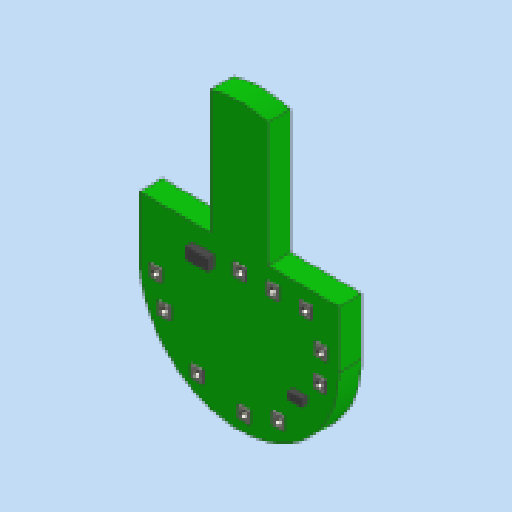
# Autodesk Inventor part: Sensor_PCB
Saved by Autodesk Inventor 2024 (Build 280153000, 153)
## iProperties
Created: 2025-02-15
Part Number: Sensor_PCB
Material: Generic
Document SubType Name: Modeling
Designer: XxPan
Density: 1 g/cm^3
Appearance: Default
Author: XxPan
Autodesk Inventor part; units mm, degrees
ref_plane "YZ Plane" through (0, 0, 0) normal (1, 0, 0) x (0, 1, 0)
ref_plane "XZ Plane" through (0, 0, 0) normal (0, 1, 0) x (-1, 0, 0)
ref_plane "XY Plane" through (0, 0, 0) normal (0, 0, 1) x (1, 0, 0)
sketch "Sketch1" plane through (0, 0, 0) normal (0, 0, 1) x (-1, 0, 0)
  line L0 (0, 0) -> (0, 6) construction
  line L1 (7, 0) -> (7, 6)
  line L2 (-7, 6) -> (-7, 0)
  arc A0 (-7, 0) -> (7, 0) centre (0, 0) ccw
  arc A1 (7, 6) -> (-7, 6) centre (0, 6) ccw
  point P0 (0, 3)
  dimension "d4" = 6
  dimension "d5" = 14
  constraints: 8 end point, 4 point on circle, 4 tangent, 2 centre point, 1 midpoint, 1 parallel, 1 vertical
  measures "d4" distance of L0.start L0.end
  measures "d5" diameter of A1
extrude "Extrusion1" add sketch "Sketch1" along normal blind 1.6
sketch "Sketch2" plane through (0, 0, 0) normal (0, 0, -1) x (-1, 0, 0)
  line L0 (-7, -6) -> (-7, 0) projected
  line L1 (-7, -2) -> (-2, -2)
  line L2 (-2, -2) -> (-2, 6.7082)
  arc A0 (7, 0) -> (-7, 0) centre (0, 0) ccw projected
  line L3 (7, -2) -> (2, -2)
  line L4 (2, -2) -> (2, 6.7082)
  line L5 (7, 0) -> (7, -6) projected
  line L6 (0, -17) -> (0, 11) construction
  line L7 (-9.8, 0) -> (9.8, 0) construction
  dimension "d6" = 4
  dimension "d7" = 2
  constraints: 8 end point, 3 point on line, 2 perpendicular, 2 point on circle, 1 horizontal, 1 other
  measures "d6" distance between parallel lines of L4 L2
  measures "d7" distance between parallel lines of L7 L1
extrude "Extrusion2" cut sketch "Sketch2" against normal up to surface (1.6 mm away)
sketch "Sketch5" plane through (0, 0, 1.6) normal (0, 0, 1) x (1, 0, 0)
  line L0 (-0.325, -2.875) -> (0.525, -2.875)
  line L1 (0.525, -2.875) -> (0.525, -3.725)
  line L2 (0.525, -3.725) -> (-0.325, -3.725)
  line L3 (-0.325, -3.725) -> (-0.325, -2.875)
  line L4 (1.975, -2.875) -> (2.825, -2.875)
  line L5 (2.825, -2.875) -> (2.825, -3.725)
  line L6 (2.825, -3.725) -> (1.975, -3.725)
  line L7 (1.975, -3.725) -> (1.975, -2.875)
  line L8 (4.275, -2.875) -> (5.125, -2.875)
  line L9 (5.125, -2.875) -> (5.125, -3.725)
  line L10 (5.125, -3.725) -> (4.275, -3.725)
  line L11 (4.275, -3.725) -> (4.275, -2.875)
  line L12 (5.375, -4.875) -> (6.225, -4.875)
  line L13 (6.225, -4.875) -> (6.225, -5.725)
  line L14 (6.225, -5.725) -> (5.375, -5.725)
  line L15 (5.375, -5.725) -> (5.375, -4.875)
  line L16 (5.275, -6.875) -> (6.125, -6.875)
  line L17 (6.125, -6.875) -> (6.125, -7.725)
  line L18 (6.125, -7.725) -> (5.275, -7.725)
  line L19 (5.275, -7.725) -> (5.275, -6.875)
  line L20 (2.375, -10.575) -> (3.225, -10.575)
  line L21 (3.225, -10.575) -> (3.225, -11.425)
  line L22 (3.225, -11.425) -> (2.375, -11.425)
  line L23 (2.375, -11.425) -> (2.375, -10.575)
  line L24 (-0.025, -11.375) -> (0.825, -11.375)
  line L25 (0.825, -11.375) -> (0.825, -12.225)
  line L26 (0.825, -12.225) -> (-0.025, -12.225)
  line L27 (-0.025, -12.225) -> (-0.025, -11.375)
  line L28 (-3.325, -10.575) -> (-2.475, -10.575)
  line L29 (-2.475, -10.575) -> (-2.475, -11.425)
  line L30 (-2.475, -11.425) -> (-3.325, -11.425)
  line L31 (-3.325, -11.425) -> (-3.325, -10.575)
  line L32 (-5.625, -7.875) -> (-4.775, -7.875)
  line L33 (-4.775, -7.875) -> (-4.775, -8.725)
  line L34 (-4.775, -8.725) -> (-5.625, -8.725)
  line L35 (-5.625, -8.725) -> (-5.625, -7.875)
  line L36 (-6.225, -5.875) -> (-5.375, -5.875)
  line L37 (-5.375, -5.875) -> (-5.375, -6.725)
  line L38 (-5.375, -6.725) -> (-6.225, -6.725)
  line L39 (-6.225, -6.725) -> (-6.225, -5.875)
  line L40 (7, -6) -> (7, -2) projected
  line L41 (7, -2) -> (2, -2) projected
  point P0 (0, 0)
  point P1 (4.7, -2.875)
  point P2 (5.125, -3.3)
  dimension "d22" = 0.85
  dimension "d23" = 0.85
  dimension "d24" = 0.85
  dimension "d25" = 0.85
  dimension "d26" = 0.85
  dimension "d27" = 0.85
  dimension "d28" = 0.85
  dimension "d29" = 0.85
  dimension "d30" = 0.85
  dimension "d31" = 0.85
  dimension "d32" = 0.85
  dimension "d33" = 0.85
  dimension "d34" = 0.85
  dimension "d35" = 0.85
  dimension "d36" = 0.85
  dimension "d37" = 0.85
  dimension "d38" = 0.85
  dimension "d39" = 0.85
  dimension "d40" = 0.85
  dimension "d41" = 0.85
  dimension "d42" = 2.3
  dimension "d43" = 2.3
  dimension "d44" = 2
  dimension "d45" = 2
  dimension "d46" = 0.8
  dimension "d47" = 2.4
  dimension "d48" = 0.1
  dimension "d49" = 2.3
  dimension "d50" = 1.3
  dimension "d51" = 1.1
  dimension "d52" = 2.9
  dimension "d53" = 3.7
  dimension "d54" = 0.8
  dimension "d55" = 3.3
  dimension "d56" = 2.3
  dimension "d57" = 2.7
  dimension "d58" = 0.6
  dimension "d59" = 2
  constraints: 80 end point, 20 parallel, 10 horizontal, 10 perpendicular, 2 collinear, 2 midpoint
  measures "d22" distance of L1.end L2.end
  measures "d23" distance of L0.end L1.end
  measures "d24" distance of L5.end L6.end
  measures "d25" distance of L4.end L5.end
  measures "d26" distance of L9.end L10.end
  measures "d27" distance of L8.end L9.end
  measures "d28" distance of L13.end L14.end
  measures "d29" distance of L12.end L13.end
  measures "d30" distance of L17.end L18.end
  measures "d31" distance of L16.end L17.end
  measures "d32" distance of L21.end L22.end
  measures "d33" distance of L20.end L21.end
  measures "d34" distance of L25.end L26.end
  measures "d35" distance of L24.end L25.end
  measures "d36" distance of L29.end L30.end
  measures "d37" distance of L28.end L29.end
  measures "d38" distance of L33.end L34.end
  measures "d39" distance of L32.end L33.end
  measures "d40" distance of L37.end L38.end
  measures "d41" distance of L36.end L37.end
  measures "d42" distance between parallel lines of L5 L1
  measures "d43" distance between parallel lines of L9 L5
  measures "d44" distance between parallel lines of L14 L10
  measures "d45" distance between parallel lines of L18 L14
  measures "d46" distance between parallel lines of L20 L24
  measures "d47" distance between parallel lines of L21 L25
  measures "d48" distance between parallel lines of L17 L13
  measures "d49" distance from line of L40 point (4.7, -2.875)
  measures "d50" distance from line of L41 point (5.125, -3.3)
  measures "d51" distance between parallel lines of L13 L9
  measures "d52" distance between parallel lines of L17 L21
  measures "d53" distance between parallel lines of L16 L20
  measures "d54" distance between parallel lines of L26 L30
  measures "d55" distance between parallel lines of L27 L31
  measures "d56" distance between parallel lines of L35 L31
  measures "d57" distance between parallel lines of L28 L32
  measures "d58" distance between parallel lines of L35 L39
  measures "d59" distance between parallel lines of L32 L36
extrude "Extrusion5" add sketch "Sketch5" along normal blind 0.1 and the other way blind 1.7
sketch "Sketch6" plane through (0, 0, 1.7) normal (0, 0, 1) x (1, 0, 0)
  line L0 (0.525, -2.875) -> (-0.325, -2.875) projected
  line L1 (2.825, -2.875) -> (1.975, -2.875) projected
  line L2 (5.125, -2.875) -> (4.275, -2.875) projected
  line L3 (6.225, -4.875) -> (5.375, -4.875) projected
  line L4 (6.125, -6.875) -> (5.275, -6.875) projected
  line L5 (3.225, -10.575) -> (2.375, -10.575) projected
  line L6 (0.825, -11.375) -> (-0.025, -11.375) projected
  line L7 (-2.475, -10.575) -> (-3.325, -10.575) projected
  line L8 (-4.775, -7.875) -> (-5.625, -7.875) projected
  line L9 (-5.375, -5.875) -> (-6.225, -5.875) projected
  line L10 (-6.225, -5.875) -> (-6.225, -6.725) projected
  line L11 (-5.625, -7.875) -> (-5.625, -8.725) projected
  line L12 (-3.325, -10.575) -> (-3.325, -11.425) projected
  line L13 (-0.025, -11.375) -> (-0.025, -12.225) projected
  line L14 (2.375, -10.575) -> (2.375, -11.425) projected
  line L15 (5.275, -6.875) -> (5.275, -7.725) projected
  line L16 (5.375, -4.875) -> (5.375, -5.725) projected
  line L17 (4.275, -2.875) -> (4.275, -3.725) projected
  point P0 (0, 0)
  point P1 (0.1, -3.3)
  point P2 (2.4, -3.3)
  point P3 (4.7, -3.3)
  point P4 (5.8, -5.3)
  point P5 (5.7, -7.3)
  point P6 (2.8, -11)
  point P7 (0.4, -11.8)
  point P8 (-2.9, -11)
  point P9 (-5.2, -8.3)
  point P10 (-5.8, -6.3)
  point P11 (0.1, -2.875)
  point P12 (2.4, -2.875)
  point P13 (4.7, -2.875)
  point P14 (5.8, -4.875)
  point P15 (5.7, -6.875)
  point P16 (2.8, -10.575)
  point P17 (0.4, -11.375)
  point P18 (-2.9, -10.575)
  point P19 (-5.2, -7.875)
  point P20 (-5.8, -5.875)
  point P21 (-6.225, -6.3)
  point P22 (-5.625, -8.3)
  point P23 (-3.325, -11)
  point P24 (-0.025, -11.8)
  point P25 (2.375, -11)
  point P26 (5.275, -7.3)
  point P27 (5.375, -5.3)
  point P28 (4.275, -3.3)
  constraints: 18 midpoint, 10 horizontal alignment, 10 vertical alignment
hole "Hole1" at (0.1, -3.3, 1.7) at (2.4, -3.3, 1.7) at (4.7, -3.3, 1.7) at (5.8, -5.3, 1.7) at (5.7, -7.3, 1.7) at (2.8, -11, 1.7) at (0.4, -11.8, 1.7) at (-2.9, -11, 1.7) at (-5.2, -8.3, 1.7) at (-5.8, -6.3, 1.7) direction (0, 0, -1) diameter 0.5 end through all
sketch "sketch3" plane through (0, 0, 1.6) normal (0, 0, 1) x (1, 0, 0)
  line L0 (-3.3, -3.2) -> (-1.7, -3.2)
  line L1 (-1.7, -3.2) -> (-1.7, -4)
  line L2 (-1.7, -4) -> (-3.3, -4)
  line L3 (-3.3, -4) -> (-3.3, -3.2)
  line L4 (-7, -2) -> (-7, -6) projected
  line L5 (-2, -2) -> (-7, -2) projected
  point P0 (0, 0)
  point P1 (-7, -4)
  point P2 (-2.5, -3.2)
  point P3 (-5, -2)
  point P4 (-3.3, -3.6)
  dimension "d12" = 1.6
  dimension "d13" = 0.8
  dimension "d20" = 4.5
  dimension "d21" = 1.6
  constraints: 8 end point, 2 midpoint, 2 parallel, 1 horizontal, 1 perpendicular
  measures "d12" distance of L1.end L2.end
  measures "d13" distance of L0.end L1.end
  measures "d20" distance from line of L4 point (-2.5, -3.2)
  measures "d21" distance from line of L5 point (-3.3, -3.6)
extrude "front 0603 res" add sketch "sketch3" along normal blind 0.5
sketch "Sketch4" plane through (0, 0, 1.6) normal (0, 0, 1) x (1, 0, 0)
  line L0 (3.7846, -8.5335) -> (4.7846, -8.5335)
  line L1 (4.7846, -8.5335) -> (4.7846, -9.0335)
  line L2 (4.7846, -9.0335) -> (3.7846, -9.0335)
  line L3 (3.7846, -9.0335) -> (3.7846, -8.5335)
  point P0 (0, 0)
  dimension "d16" = 1
  dimension "d17" = 0.5
  constraints: 8 end point, 2 parallel, 1 horizontal, 1 perpendicular
  measures "d16" distance of L1.end L2.end
  measures "d17" distance of L0.end L1.end
extrude "front 0402 res" add sketch "Sketch4" along normal blind 0.4
sketch "Sketch7" plane through (0, 0, 0) normal (0, 0, -1) x (-1, 0, 0)
  line L0 (1.075, -7.15) -> (2.325, -7.15)
  line L1 (2.325, -7.15) -> (2.325, -9.15)
  line L2 (2.325, -9.15) -> (1.075, -9.15)
  line L3 (1.075, -9.15) -> (1.075, -7.15)
  line L4 (7, -2) -> (7, -6) projected
  arc A0 (-7, -6) -> (7, -6) centre (0, -6) ccw projected
  point P0 (0, 0)
  point P1 (1.7, -7.15)
  point P2 (0, -13)
  point P3 (2.325, -8.15)
  dimension "d71" = 1.25
  dimension "d72" = 2
  dimension "d73" = 5.3
  dimension "d74" = 4.85
  constraints: 8 end point, 2 midpoint, 2 parallel, 1 horizontal, 1 perpendicular, 1 point on circle
  measures "d71" distance of L1.end L2.end
  measures "d72" distance of L0.end L1.end
  measures "d73" distance from line of L4 point (1.7, -7.15)
  measures "d74" vertical distance of point (0, -13) point (2.325, -8.15)
extrude "back 0805 cap" add sketch "Sketch7" along normal blind 1.25
sketch "Sketch8" plane through (0, 0, 0) normal (0, 0, -1) x (-1, 0, 0)
  line L0 (0.4, -5.3) -> (2, -5.3)
  line L1 (2, -5.3) -> (2, -6.1)
  line L2 (2, -6.1) -> (0.4, -6.1)
  line L3 (0.4, -6.1) -> (0.4, -5.3)
  line L4 (7, -2) -> (7, -6) projected
  line L5 (7, -2) -> (2, -2) projected
  point P0 (0, 0)
  point P1 (1.2, -5.3)
  point P2 (2, -5.7)
  dimension "d77" = 1.6
  dimension "d78" = 0.8
  dimension "d79" = 5.8
  dimension "d80" = 3.7
  constraints: 8 end point, 2 midpoint, 2 parallel, 1 horizontal, 1 perpendicular
  measures "d77" distance of L1.end L2.end
  measures "d78" distance of L0.end L1.end
  measures "d79" distance from line of L4 point (1.2, -5.3)
  measures "d80" distance from line of point (2, -5.7) L5
extrude "back 0603 cap" add sketch "Sketch8" along normal blind 0.8
sketch "Sketch9" plane through (0, 0, 0) normal (0, 0, -1) x (-1, 0, 0)
  line L0 (-0.05, -7.15) -> (0.45, -7.15)
  line L1 (0.45, -7.15) -> (0.45, -8.15)
  line L2 (0.45, -8.15) -> (-0.05, -8.15)
  line L3 (-0.05, -8.15) -> (-0.05, -7.15)
  line L4 (1.075, -9.15) -> (2.325, -9.15) projected
  line L5 (1.075, -7.15) -> (1.075, -9.15) projected
  point P0 (0, 0)
  point P1 (1.7, -9.15)
  point P2 (0.2, -8.15)
  point P3 (0.45, -7.65)
  point P4 (1.075, -8.15)
  dimension "d83" = 0.5
  dimension "d84" = 1
  dimension "d85" = 1.5
  dimension "d86" = 0.5
  constraints: 8 end point, 4 midpoint, 2 parallel, 1 horizontal, 1 perpendicular
  measures "d83" distance of L1.end L2.end
  measures "d84" distance of L0.end L1.end
  measures "d85" horizontal distance of point (1.7, -9.15) point (0.2, -8.15)
  measures "d86" vertical distance of point (0.45, -7.65) point (1.075, -8.15)
extrude "back 0402 cap" add sketch "Sketch9" along normal blind 0.5
sketch "Sketch10" plane through (0, 0, 0) normal (0, 0, -1) x (-1, 0, 0)
  line L0 (-2.8, -7.25) -> (-2, -7.25)
  line L1 (-2, -7.25) -> (-2, -8.85)
  line L2 (-2, -8.85) -> (-2.8, -8.85)
  line L3 (-2.8, -8.85) -> (-2.8, -7.25)
  line L4 (0.45, -7.15) -> (-0.05, -7.15) projected
  line L5 (-0.05, -7.15) -> (-0.05, -8.15) projected
  point P0 (0, 0)
  point P1 (0.2, -7.15)
  point P2 (-2.4, -7.25)
  point P3 (0.2, -7.15)
  point P4 (-0.05, -7.65)
  point P5 (-2, -8.05)
  dimension "d89" = 0.8
  dimension "d90" = 1.6
  dimension "d92" = 2.6
  dimension "d93" = 0.4
  constraints: 8 end point, 5 midpoint, 2 parallel, 1 horizontal, 1 perpendicular
  measures "d89" distance of L1.end L2.end
  measures "d90" distance of L0.end L1.end
  measures "d92" horizontal distance of point (0.2, -7.15) point (-2.4, -7.25)
  measures "d93" vertical distance of point (-0.05, -7.65) point (-2, -8.05)
extrude "back 0603 res" add sketch "Sketch10" along normal blind 0.8
body "Solid1"
